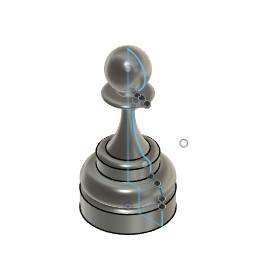
pawn (Autodesk Fusion 360 design; units mm, degrees)
Autodesk Fusion 360 part; units mm, degrees
sketch "Sketch1" plane through (0, 0, 0) normal (0, 1, 0) x (1, 0, 0)
  line L0 (4.127, 0) -> (12.7, 0)
  line L1 (0, -8.1) -> (0, -50.8)
  line L2 (4.127, -8.1) -> (4.127, 0)
  line L3 (4.127, -8.1) -> (0, -8.1)
  line L4 (12.7, 0) -> (12.7, -6.35)
  spline S0 degree 5 poles (12.7, -6.35) (12.540347, -6.437114) (12.244903, -6.604312) (11.873327, -6.834016) (11.521626, -7.097954) (11.318881, -7.360397) (11.338314, -7.566884) (11.546614, -7.741182) (11.880766, -7.92652) (12.256592, -8.177168) (12.586876, -8.541968) (12.795075, -9.051819) (12.833746, -9.701765) (12.692205, -10.446184) (12.384964, -11.217988) (11.944919, -11.942084) (11.415148, -12.550985) (10.841724, -12.999356) (10.266175, -13.27996) (9.718479, -13.438247) (9.219166, -13.548653) (8.868582, -13.664055) (8.636051, -13.79592) (8.494772, -13.907953) (8.427569, -13.97) knots 0 0 0 0 0 0 0.05 0.1 0.15 0.2 0.25 0.3 0.35 0.4 0.45 0.5 0.55 0.6 0.65 0.7 0.75 0.8 0.85 0.9 0.95 1 1 1 1 1 1
  line L5 (9.283387, -13.179847) -> (7.57175, -14.760154)
  spline S1 degree 5 poles (1.947187, -33.385045) (1.956572, -33.483951) (1.977063, -33.685801) (2.01295, -34.00071) (2.074709, -34.434176) (2.192832, -34.943425) (2.371983, -35.35619) (2.622791, -35.628945) (2.946665, -35.747223) (3.307395, -35.782693) (3.685406, -35.81064) (4.094457, -35.856142) (4.552987, -35.926772) (5.06597, -36.007474) (5.619113, -36.0799) (6.127615, -36.111102) (6.518442, -36.113185) (6.791399, -36.147804) (6.967622, -36.257863) (7.081601, -36.455526) (7.153497, -36.615012) (7.171237, -36.730186) (7.108655, -36.86104) (6.940806, -37.046392) (6.656984, -37.262925) (6.260302, -37.460615) (5.773435, -37.591106) (5.234911, -37.625433) (4.71595, -37.60712) (4.28735, -37.613103) (3.954761, -37.630653) (3.700462, -37.642691) (3.487455, -37.629722) (3.284375, -37.639029) (3.068122, -37.742064) (2.808309, -37.928911) (2.544461, -38.123806) (2.305908, -38.278169) (2.12771, -38.382215) (2.03382, -38.434514) knots 0 0 0 0 0 0 0.02857143 0.05714286 0.08571429 0.11428571 0.14285714 0.17142857 0.2 0.22857143 0.25714286 0.28571429 0.31428571 0.34285714 0.37142857 0.4 0.42857143 0.45714286 0.48571429 0.51428571 0.54285714 0.57142857 0.6 0.62857143 0.65714286 0.68571429 0.71428571 0.74285714 0.77142857 0.8 0.82857143 0.85714286 0.88571429 0.91428571 0.94285714 0.97142857 1 1 1 1 1 1
  line L6 (1.817127, -32.014396) -> (2.077247, -34.755695)
  line L7 (2.06818, -35.484547) -> (3.775207, -35.95082)
  line L8 (3.943882, -35.904704) -> (7.232118, -36.231296)
  line L9 (6.556734, -35.627964) -> (7.513825, -37.143894)
  line L10 (6.858, -37.592) -> (3.467388, -37.635994)
  line L11 (3.733769, -37.487616) -> (0.33387, -39.381412)
  line L12 (8.427569, -13.97) -> (8.427569, -17.815821)
  arc A0 (5.887569, -19.085821) -> (8.427569, -17.815821) centre (6.305857, -16.747397) ccw
  arc A1 (5.887569, -19.085821) -> (1.947187, -33.385045) centre (20.845636, -30.900288) ccw
  arc A2 (0, -50.8) -> (2.03382, -38.434514) centre (0, -44.45) ccw
  line L13 (4.197727, -37.613997) -> (2.737049, -37.657991)
  point P0 (11.43, -7.62)
  point P1 (12.7, -8.89)
  point P2 (10.868259, -12.940271)
  point P3 (2.921694, -35.717684)
  point P4 (7.03528, -36.385929)
  point P5 (7.112, -36.83)
  point P6 (5.162694, -37.613997)
  point P7 (5.588, -36.068)
  point P8 (3.467388, -37.635994)
  dimension "d1" = 12.7
  dimension "d2" = 50.8
  dimension "d5" = 6.35
  dimension "d7" = 12.7
  dimension "d9" = 4.127
  dimension "d10" = 8.1
  constraint horizontal L0
  constraint perpendicular L0 L1
  constraint perpendicular L0 L2
  constraint perpendicular L1 L3
  constraint perpendicular L0 L4
  constraint midpoint P7 L8
  constraint vertical L12
  measures "d1" distance of origin L0.end
  measures "d2" distance of origin L1.end
  measures "d5" distance of L0.end L4.end
  measures "d7" diameter of A2
  measures "d9" distance of L1.start L2.start
  measures "d10" distance of L0.start L2.start
revolve "Revolve1" add sketch "Sketch1" angle 360 about axis through (0, 0, 8.1) along (0, 0, 1) contours L0 L1 L2 L3 L4 S0 S1 L8 L10 L11 L12 A0 A1 A2 | S1 L8 picked at (6.56431, -5.111544) picked at (6.578911, -36.145702)
equation "d2 = 2\""
